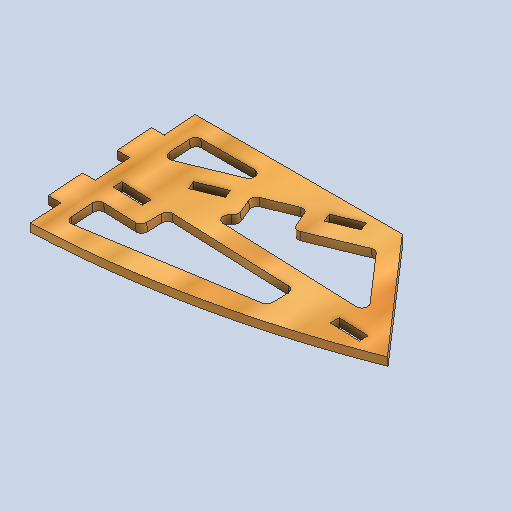
# Autodesk Inventor part: bulkhead_sponson_break
Saved by Autodesk Inventor 2022 (Build 260153070, 153G)
## iProperties
Created: 2021-04-25
Part Number: bulkhead_sponson_break
Material: Plywood, Sheathing, Glazed
Document SubType Name: Modeling
Designer: kardo
Density: 0.75 g/cm^3
Appearance: Plywood - New(2)
Mass: 2.06355 g
Surface Area: 37.6832 cm^2
Volume: 2.7514 cm^3
Author: kardo
Autodesk Inventor part; units mm, degrees
ref_plane "YZ Plane" through (0, 0, 0) normal (1, 0, 0) x (0, 1, 0)
ref_plane "XZ Plane" through (0, 0, 0) normal (0, 1, 0) x (-1, 0, 0)
ref_plane "XY Plane" through (0, 0, 0) normal (0, 0, 1) x (1, 0, 0)
derived "frame_outline.ipt"
sketch "bh_sponson_break" plane through (81, 130.35, 9.115) normal (0, -0.9975641, -0.0697565) x (1, 0, 0)
  line L0 (75.1695, 26.4514) -> (52.5, 0) construction
  line L1 (52.5, 0) -> (0, 0) construction
  line L2 (73.8074, 26.0914) -> (52.132, 0.8)
  line L3 (52.132, 0.8) -> (0, 0.8)
  line L4 (0, 0.8) -> (0, 40.103)
  spline S0 degree 2 poles (75.1695, 26.4514) (38.4998, 39.7466) (0, 40.9033) knots 0 0 0 1 1 1
  spline S1 degree 3 poles (0, 40.103) (4.1988, 39.9764) (11.5178, 39.5648) (19.8248, 38.7141) (26.0304, 37.9132) (30.1551, 37.2978) (35.2958, 36.4267) (39.396, 35.6483) (44.506, 34.5735) (48.5818, 33.6322) (53.6612, 32.3536) (57.7126, 31.2493) (62.7615, 29.7669) (67.7953, 28.1827) (71.806, 26.8066) (73.8074, 26.0914) knots 0.014896 0.014896 0.014896 0.014896 0.179028 0.302127 0.34316 0.425226 0.466258 0.548324 0.589357 0.671423 0.712456 0.794522 0.835555 0.917621 0.999687 0.999687 0.999687 0.999687
  point P0 (-81, 0)
  point P1 (3, 18.694)
  point P2 (3, 23.7222)
  point P3 (0, 32.7227)
  point P4 (0, 24.542)
  point P5 (0, 16.3613)
  point P6 (0, 8.1807)
extrude "Extrusion1" add sketch "bh_sponson_break" along normal blind 2
sketch "Sketch4" plane through (81, 130.2942, 9.913) normal (0, 0.9975641, 0.0697565) x (1, 0, 0)
  line L0 (0, -31.9227) -> (3, -31.9227)
  line L1 (3, -31.9227) -> (3, -39.1939)
  spline S0 degree 3 poles (73.8074, -25.2914) (71.806, -26.0066) (67.7953, -27.3827) (62.7615, -28.9669) (57.7126, -30.4493) (53.6612, -31.5536) (48.5818, -32.8322) (44.506, -33.7735) (39.396, -34.8483) (35.2958, -35.6267) (30.1551, -36.4978) (26.0304, -37.1132) (19.8248, -37.9141) (11.5178, -38.7648) (4.1988, -39.1764) (0, -39.303) knots 0 0 0 0 0.083333 0.166667 0.208333 0.291667 0.333333 0.416667 0.458333 0.541667 0.583333 0.666667 0.708333 0.833333 1 1 1 1 projected
  line L2 (0, 0) -> (52.132, 0) projected
  line L3 (0, -7.3807) -> (3, -7.3807)
  line L4 (3, -7.3807) -> (3, 0)
  line L5 (0, 0) -> (52.132, 0) projected
  line L6 (0, -15.5613) -> (3, -15.5613)
  line L7 (3, -15.5613) -> (3, -23.742)
  line L8 (3, -23.742) -> (0, -23.742)
  line L9 (0, -31.9227) -> (0, -39.303)
  line L10 (0, -31.9227) -> (0, -23.742)
  line L11 (0, -15.5613) -> (0, -7.3807)
  line L12 (0, 0) -> (0, -7.3807)
  line L13 (0, -15.5613) -> (0, -23.742)
  point P0 (-81, 0.8)
  point P1 (3, 0)
  point P2 (0, -31.9227)
  point P3 (0, -23.742)
  point P4 (0, -7.3807)
  point P5 (0, -15.5613)
  dimension "d39" = 3
  constraints: 24 end point, 6 collinear, 5 point on line, 4 perpendicular, 1 parallel, 2 other
  measures "d39" distance of L3.start L3.end
extrude "Extrusion4" cut sketch "Sketch4" against normal through all both and the other way through all
sketch "Sketch2" plane through (81, 130.2942, 9.913) normal (0, 0.9975641, 0.0697565) x (1, 0, 0)
  line L0 (67.233, -25.3512) -> (67.3086, -23.3527)
  line L1 (67.3086, -23.3527) -> (60.1716, -23.0828)
  line L2 (60.1716, -23.0828) -> (60.096, -25.0813)
  line L3 (13.7055, -23.327) -> (13.7811, -21.3285)
  line L4 (13.7811, -21.3285) -> (6.6441, -21.0586)
  line L5 (6.6441, -21.0586) -> (6.5685, -23.0571)
  line L6 (75.1695, -25.6514) -> (74.37, -25.6211) construction
  line L7 (74.37, -25.6211) -> (3, -22.9222)
  line L8 (52.5, 0.8) -> (51.7516, 0.5174) construction
  line L9 (51.7516, 0.5174) -> (3, -17.894)
  line L10 (15.6754, -13.107) -> (16.382, -14.978)
  line L11 (16.382, -14.978) -> (22.7197, -12.5846)
  line L12 (22.7197, -12.5846) -> (22.0131, -10.7135)
  line L13 (45.4139, -1.8761) -> (46.1205, -3.7471)
  line L14 (46.1205, -3.7471) -> (39.7828, -6.1406)
  line L15 (39.7828, -6.1406) -> (39.0762, -4.2696)
  point P0 (-81, 0.8)
  dimension "d6" = 0.8
  dimension "d7" = 71.421
  dimension "d8" = 7.1421
  dimension "d9" = 7.1421
  dimension "d10" = 2
  dimension "d11" = 7.1421
  dimension "d12" = 3.5711
  dimension "d13" = 0.8
  dimension "d14" = 52.1123
  dimension "d15" = 6.7746
  dimension "d16" = 6.7746
  dimension "d17" = 2
  dimension "d18" = 6.7746
  dimension "d19" = 13.5492
  constraints: 32 end point, 8 perpendicular, 8 point on line, 4 collinear, 3 parallel
  measures "d6" distance of L6.start L6.end
  measures "d7" distance of L6.end L7.end
  measures "d8" distance of L0.end L1.end
  measures "d9" distance of L3.end L4.end
  measures "d10" distance of L1.end L2.end
  measures "d11" distance from line of L6.end L0
  measures "d12" distance from line of L7.end L5
  measures "d13" distance of L8.start L8.end
  measures "d14" distance of L8.end L9.end
  measures "d15" distance of L13.end L14.end
  measures "d16" distance of L10.end L11.end
  measures "d17" distance of L14.end L15.end
  measures "d18" distance from line of L8.end L13
  measures "d19" distance from line of L9.end L10
extrude "Extrusion2" cut sketch "Sketch2" against normal through all
sketch "Sketch3" plane through (81, 130.2942, 9.913) normal (0, 0.9975641, 0.0697565) x (1, 0, 0)
  line L0 (60.1716, -23.0828) -> (67.3086, -23.3527) projected
  line L1 (6.6441, -21.0586) -> (13.7811, -21.3285) projected
  line L2 (22.7197, -12.5846) -> (16.382, -14.978) projected
  line L3 (46.1205, -3.7471) -> (39.7828, -6.1406) projected
  line L4 (39.0762, -4.2696) -> (45.4139, -1.8761) projected
  line L5 (15.6754, -13.107) -> (22.0131, -10.7135) projected
  line L6 (13.7055, -23.327) -> (6.5685, -23.0571) projected
  line L7 (67.233, -25.3512) -> (60.096, -25.0813) projected
  line L8 (52.132, 0) -> (73.8074, -25.2914) projected
  line L9 (0, 0) -> (52.132, 0) projected
  line L10 (63.3179, -19.1989) -> (20.7862, -17.5905)
  line L11 (20.7862, -17.5905) -> (51.8767, -5.849)
  line L12 (51.8767, -5.849) -> (63.3179, -19.1989)
  line L13 (7, -27.0763) -> (7, -34.9993)
  line L14 (7, -34.9993) -> (48.8211, -28.6578)
  line L15 (48.8211, -28.6578) -> (7, -27.0763)
  line L16 (48.8211, -28.6578) -> (49.4208, -32.6126) construction
  line L17 (7, -34.9993) -> (7.5997, -38.9541) construction
  line L18 (28.4682, -4) -> (7, -12.1076)
  line L19 (7, -12.1076) -> (7, -4)
  line L20 (7, -4) -> (28.4682, -4)
  line L21 (48.8211, -28.6578) -> (49.0479, -22.6621)
  line L22 (49.0479, -22.6621) -> (17.7782, -21.4796)
  line L23 (17.7782, -21.4796) -> (17.5515, -27.4753)
  line L24 (13.7811, -21.3285) -> (13.7055, -23.327) projected
  line L25 (37.4539, -11.2958) -> (35.3341, -5.6828)
  line L26 (35.3341, -5.6828) -> (25.7552, -9.3003)
  line L27 (25.7552, -9.3003) -> (27.875, -14.9134)
  line L28 (39.7828, -6.1406) -> (39.0762, -4.2696) projected
  line L29 (22.0131, -10.7135) -> (22.7197, -12.5846) projected
  line L30 (3, -31.9227) -> (3, -39.1939) projected
  line L31 (3, -15.5613) -> (3, -23.742) projected
  line L32 (3, 0) -> (3, -7.3807) projected
  point P0 (-81, 0.8)
  dimension "d22" = 4
  dimension "d23" = 4
  dimension "d24" = 4
  dimension "d25" = 4
  dimension "d27" = 4
  dimension "d28" = 4
  dimension "d29" = 4
  dimension "d33" = 4
  dimension "d34" = 4
  dimension "d35" = 4
  dimension "d36" = 4
  dimension "d37" = 4
  dimension "d42" = 4
  dimension "d43" = 4
  constraints: 34 end point, 9 parallel, 6 perpendicular, 3 point on line, 3 other
  measures "d22" distance between parallel lines of L8 L12
  measures "d23" distance between parallel lines of L0 L10
  measures "d24" distance between parallel lines of L3 L11
  measures "d25" distance between parallel lines of L6 L15
  measures "d27" distance of L13.end L17.end
  measures "d28" distance between parallel lines of L5 L18
  measures "d29" distance between parallel lines of L9 L20
  measures "d33" distance between parallel lines of L22 L10
  measures "d34" distance between parallel lines of L24 L23
  measures "d35" distance between parallel lines of L25 L28
  measures "d36" distance between parallel lines of L27 L29
  measures "d37" distance between parallel lines of L18 L26
  measures "d42" distance between parallel lines of L30 L13
  measures "d43" distance between parallel lines of L32 L19
extrude "Extrusion3" cut sketch "Sketch3" against normal through all
fillet "Fillet1" radius 1.3333 16 edges at (88, 126.8552, 44.7573) (88, 128.452, 21.9214) (98.5515, 127.38, 37.2517) (88, 129.0176, 13.8335) (109.4682, 129.0176, 13.8335) (130.0479, 127.7158, 32.4502) (116.3341, 128.9002, 15.5122) (118.4539, 128.5087, 21.1116) (108.875, 128.2563, 24.7203) (106.7552, 128.6479, 19.1209) (132.8767, 128.8886, 15.678) (144.3179, 127.9574, 28.9954) (101.7862, 128.0696, 27.3909) (129.8211, 127.2976, 38.4313) (98.7782, 127.7983, 31.2705) (88, 127.4079, 36.8536)
equation "\"d1\" = bulkhead_thickness"
equation "\"d39\" = stringer_thickness"
equation "\"d6\" = surface_thickness"
equation "\"d8\" = 0.1 * d7"
equation "\"d9\" = 0.1 * d7"
equation "\"d10\" = bulkhead_thickness"
equation "\"d11\" = d8"
equation "\"d12\" = 0.5 * d9"
equation "\"d13\" = surface_thickness"
equation "\"d15\" = 0.13 * d14"
equation "\"d16\" = 0.13 * d14"
equation "\"d17\" = bulkhead_thickness"
equation "\"d18\" = d15"
equation "\"d19\" = 2 * d16"
equation "\"d22\" = inset"
equation "\"d23\" = inset"
equation "\"d24\" = inset"
equation "\"d25\" = inset"
equation "\"d27\" = inset"
equation "\"d28\" = inset"
equation "\"d29\" = inset"
equation "\"d33\" = inset"
equation "\"d34\" = inset"
equation "\"d35\" = inset"
equation "\"d36\" = inset"
equation "\"d37\" = inset"
equation "\"d42\" = inset"
equation "\"d43\" = inset"
equation "\"d38\" = 0.333333 * inset"
equation "\"bulkhead_thickness\" = 2"
equation "\"stringer_thickness\" = 3"
equation "\"surface_thickness\" = 0.8"
equation "\"inset\" = 4"
body "Solid1"
